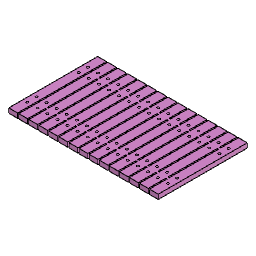
0_Schwellenband_Holz_K_Modul_System_v2 (Autodesk Fusion 360 design; units mm, degrees)
Autodesk Fusion 360 part; units mm, degrees
sketch "Skizze1" plane through (0, 0, 0) normal (0, 0, 1) x (1, 0, 0)
  line L0 (0, 29) -> (0, -29)
  line L1 (0, -29) -> (5.75, -29)
  line L2 (5.75, -29) -> (5.75, 29)
  line L3 (5.75, 29) -> (0, 29)
  line L4 (2.875, 29) -> (2.875, -29) construction
  line L5 (0, 0) -> (5.75, 0) construction
  circle A0 centre (2.875, 19.75) radius 0.75
  circle A1 centre (2.875, 13.75) radius 0.75
  circle A2 centre (2.875, -19.75) radius 0.75
  circle A3 centre (2.875, -13.75) radius 0.75
  dimension "d1" = 58
  dimension "d2" = 5.75
  dimension "d9" = 1.5
  dimension "d10" = 1.5
  dimension "d11" = 6
  dimension "d12" = 13.75
  constraint perpendicular L0 L1
  constraint perpendicular L1 L2
  constraint perpendicular L0 L3
  constraint vertical L0
  constraint midpoint L5.start L0
  constraint midpoint L3 L4.start
  constraint midpoint L1 L4.end
  constraint coincident L5.start origin
  constraint midpoint L2 L5.end
  constraint coincident L4 A0.centre
  constraint coincident L4 A1.centre
  constraint symmetric L5 A0 A2
  constraint symmetric L5 A1 A3
  measures "d1" distance of L0.start L0.end
  measures "d2" distance of L0.start L2.end
  measures "d9" diameter of A0
  measures "d10" diameter of A1
  measures "d11" distance of A0.centre A1.centre
  measures "d12" distance of L5 A1.centre
extrude "Extrusion1" add sketch "Skizze1" along normal blind 3 makes body 1
pattern_linear "R-Anordnung1" count 15 spacing 6.55 along (1, 0, 0) of bodies 1 makes body 2 at (9.4346, 26.1665, 0) makes body 3 at (15.9846, 26.1665, 0) makes body 4 at (22.5346, 26.1665, 0) makes body 5 at (29.0846, 26.1665, 0) makes body 6 at (35.6346, 26.1665, 0) makes body 7 at (42.1846, 26.1665, 0) makes body 8 at (48.7346, 26.1665, 0) makes body 9 at (55.2846, 26.1665, 0) makes body 10 at (61.8346, 26.1665, 0) makes body 11 at (68.3846, 26.1665, 0) makes body 12 at (74.9346, 26.1665, 0) makes body 13 at (81.4846, 26.1665, 0) makes body 14 at (88.0346, 26.1665, 0) makes body 15 at (94.5846, 26.1665, 0)
sketch "Skizze2" plane through (0, 0, 0) normal (0, 0, 1) x (1, 0, 0)
  line L0 (12.3, -29) -> (12.3, 29)
  circle A0 centre (9.425, 13.75) radius 0.75
  circle A1 centre (9.425, 19.75) radius 0.75
  line L1 (12.3, 0) -> (91.7, 0) construction
  line L2 (9.425, 19.75) -> (91.7, 19.75) construction
  line L3 (9.425, 13.75) -> (91.7, 13.75) construction
  line L4 (12.3, 16.05) -> (91.7, 16.05)
  line L5 (12.3, 17.45) -> (91.7, 17.45)
  line L6 (52, 17.45) -> (52, 19.75) construction
  line L7 (52, 16.05) -> (52, 13.75) construction
  line L8 (12.3, -16.05) -> (91.7, -16.05)
  line L9 (12.3, -17.45) -> (91.7, -17.45)
  line L10 (91.7, 29) -> (91.7, -29)
  dimension "d20" = 1.4
  constraint midpoint L0 L1.start
  constraint coincident A1.centre L2.start
  constraint coincident A0.centre L3.start
  constraint coincident L0 L4.start
  constraint coincident L0 L5.start
  constraint midpoint L5 L6.start
  constraint coincident L2 L6.end
  constraint perpendicular L2 L6
  constraint midpoint L4 L7.start
  constraint coincident L3 L7.end
  constraint perpendicular L3 L7
  constraint equal L6 L7
  constraint symmetric L1 L4.start L8.start
  constraint symmetric L1 L4.end L8.end
  constraint symmetric L1 L5.start L9.start
  constraint symmetric L1 L5.end L9.end
  constraint coincident L2.end L10
  constraint coincident L5.end L10
  constraint coincident L4.end L10
  constraint coincident L3.end L10
  constraint perpendicular L2 L10
  constraint perpendicular L5 L10
  constraint perpendicular L3 L10
  constraint midpoint L1.end L10
  measures "d20" distance of L4 L5
extrude "Extrusion2" add sketch "Skizze2" along normal blind 3 contours L0 L8 L9 L10 | L0 L4 L5 L10 bodies 3 2 4 5 6 7 8 9 10 11 12 13 14 15
equation "d1 = Schwellen_Länge"
equation "d2 = Schwellen_Breite"
equation "Kleineisen_Bohrungsdurchmesser = 1.5 mm"
equation "Schwellen_Länge = 58 mm"
equation "Schwellen_Breite = 5.75 mm"
equation "Spurweite = 32 mm"
equation "Schienenkopf_Breite = Hegob_Schienenkopf_Breite"
equation "Kleineisen_Lochabstand = 6 mm"
equation "d9 = Kleineisen_Bohrungsdurchmesser"
equation "d10 = Kleineisen_Bohrungsdurchmesser"
equation "d11 = Kleineisen_Lochabstand"
equation "d12 = ( Spurweite / 2 ) - ( Kleineisen_Lochabstand / 2 ) + ( Schienenkopf_Breite / 2 )"
equation "Schwellen_Höhe = 3 mm"
equation "d14 = Schwellen_Höhe"
equation "d18 = 0.8 mm + Schwellen_Breite"
equation "d21 = Schwellen_Höhe"
equation "Hassler_Schienenkopf_Breite = 1.6 mm" comment "mit Toleranz"
equation "Hegob_Schienenkopf_Breite = 1.5 mm" comment "mit Toleranz"
